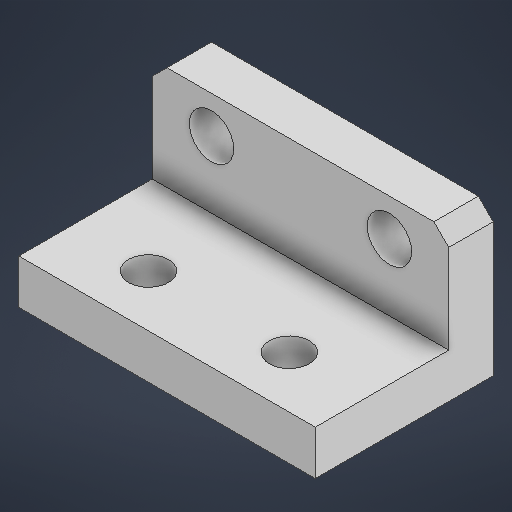
# Autodesk Inventor part: LimitSwitch_TopHolder
Saved by Autodesk Inventor 2025.2 (Build 292293000, 293)
## iProperties
Created: 2025-07-03
Part Number: LimitSwitch_TopHolder
Material: Generic
Document SubType Name: Modeling
Designer: Tiago
Density: 1 g/cm^3
Appearance: Default
Author: Tiago
Autodesk Inventor part; units mm, degrees
ref_plane "YZ Plane" through (0, 0, 0) normal (1, 0, 0) x (0, 1, 0)
ref_plane "XZ Plane" through (0, 0, 0) normal (0, 1, 0) x (-1, 0, 0)
ref_plane "XY Plane" through (0, 0, 0) normal (0, 0, 1) x (1, 0, 0)
sketch "Sketch1" plane through (0, 0, 0) normal (0, 0, 1) x (1, 0, 0)
  line L0 (-10, -5) -> (10, -5)
  line L1 (10, -5) -> (10, 5)
  line L2 (10, 5) -> (-10, 5)
  line L3 (-10, 5) -> (-10, -5)
  circle A0 centre (-6, 2.5) radius 1.5
  circle A1 centre (6, 2.5) radius 1.5
  line L4 (-10, -5) -> (10, -5)
  line L5 (10, -5) -> (10, -2)
  line L6 (10, -2) -> (-10, -2)
  line L7 (-10, -2) -> (-10, -5)
  point P0 (0, 0)
  point P1 (0, 5)
  point P2 (-10, 0)
  dimension "d0" = 10
  dimension "d1" = 20
  dimension "d2" = 3
  dimension "d3" = 3
  dimension "d4" = 12
  dimension "d5" = 6
  dimension "d6" = 2.5
  dimension "d7" = 3
  constraints: 16 end point, 4 parallel, 2 centre point, 2 horizontal, 2 horizontal alignment, 2 midpoint, 2 perpendicular, 1 point on line, 1 vertical alignment
  measures "d0" distance of L0.end L1.end
  measures "d1" distance of L0.start L0.end
  measures "d2" diameter of A1
  measures "d3" diameter of A0
  measures "d4" distance of A1.centre A0.centre
  measures "d5" horizontal distance of point (0, 0) A1.centre
  measures "d6" vertical distance of A1.centre point (0, 0)
  measures "d7" distance between parallel lines of L0 L6
extrude "Extrusion1" add sketch "Sketch1" along normal blind 3 contours L3 L2 L1 L6
extrude "Extrusion2" add sketch "Sketch1" along normal blind 12 contours L3 L6 L1 L0
sketch "Sketch2" plane through (-10, -5, 0) normal (0, -1, 0) x (1, 0, 0)
  line L0 (20, 0) -> (0, 0) projected
  line L1 (0, 0) -> (0, 12) projected
  line L2 (0, 12) -> (20, 12) projected
  line L3 (20, 12) -> (20, 0) projected
  circle A0 centre (5.25, 8.5) radius 1.35
  circle A1 centre (14.75, 8.5) radius 1.35
  point P0 (10, 0)
  dimension "d13" = 9.5
  dimension "d14" = 5.25
  dimension "d15" = 2.7
  dimension "d16" = 2.7
  dimension "d17" = 3.5
  constraints: 2 centre point, 1 horizontal alignment
  measures "d13" distance of A1.centre A0.centre
  measures "d14" distance from line of A1.centre L3
  measures "d15" diameter of A1
  measures "d16" diameter of A0
  measures "d17" distance from line of L2 A0.centre
extrude "Extrusion3" cut sketch "Sketch2" against normal up to surface (3 mm away) contours A0 | A1
chamfer "Chamfer1" distance 1 angle 45 2 edges at (10, 5, 1.5) (-10, 5, 1.5)
body "Solid1"
